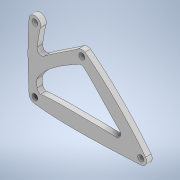
# Autodesk Inventor part: Bracket Concept MK2
Saved by Autodesk Inventor 2021 (Build 250183000, 183)
## iProperties
Created: 2021-05-11
Part Number: Bracket Concept MK2
Material: Generic
Document SubType Name: Modeling
Designer: Jawal
Density: 1 g/cm^3
Appearance: Default
Author: Jawal
Autodesk Inventor part; units mm, degrees
ref_plane "YZ Plane" through (0, 0, 0) normal (1, 0, 0) x (0, 1, 0)
ref_plane "XZ Plane" through (0, 0, 0) normal (0, 1, 0) x (-1, 0, 0)
ref_plane "XY Plane" through (0, 0, 0) normal (0, 0, 1) x (1, 0, 0)
sketch "Sketch1" plane through (0, 0, 0) normal (0, 0, 1) x (1, 0, 0)
  line L0 (-110, 70) -> (110, 70) construction
  line L1 (110, 70) -> (110, -70) construction
  line L2 (110, -70) -> (-110, -70) construction
  line L3 (-110, -70) -> (-110, 70) construction
  circle A0 centre (-90, 55) radius 5
  circle A1 centre (-90, -55) radius 5
  circle A2 centre (90, -55) radius 5
  circle A3 centre (-10, 45) radius 5
  line L4 (-67, 0) -> (-42, 0) construction
  line L5 (-42, 0) -> (-42, -30) construction
  line L6 (-42, -30) -> (-67, -30) construction
  line L7 (-67, -30) -> (-67, 0) construction
  circle A4 centre (-54.5, -11) radius 10 construction
  circle A5 centre (-63.5044, -24.4163) radius 3 construction
  circle A6 centre (-57.3559, -26.4695) radius 3 construction
  circle A7 centre (-51.263, -24.6531) radius 3 construction
  circle A8 centre (-45.3418, -26.5938) radius 3 construction
  arc A9 (-80.8676, 50.9258) -> (-100, 55) centre (-90, 55) ccw
  arc A10 (-4.8937, 53.598) -> (-15.7422, 53.187) centre (-10, 45) ccw
  arc A11 (90.4874, -64.9881) -> (88.2039, -45.1626) centre (90, -55) ccw
  line L8 (-100, 55) -> (-102.0827, 28.5336) construction
  line L9 (-102.0827, 28.5336) -> (-102.0827, 6.1317) construction
  line L10 (-102.0827, 6.1317) -> (-102.0827, -9.3012) construction
  line L11 (-102.0827, -9.3012) -> (-100, -55) construction
  spline S0 degree 4 poles (-100, 55) (-102.0827, 28.5336) (-102.0827, 6.1317) (-102.0827, -9.3012) (-100, -55) knots 1 1 1 1 1 2 2 2 2 2
  line L12 (-80.5098, 51.8478) -> (-81.3111, 50.3761) construction
  line L13 (-33.5621, 40.6884) -> (-15.7422, 53.187) construction
  spline S1 degree 3 poles (-74.3051, 13.1026) (-63.5044, 21.906) (-33.5621, 40.6884) (-15.7422, 53.187) knots 1.047287 1.047287 1.047287 1.047287 2 2 2 2
  line L14 (-90, -65) -> (-53.427, -70) construction
  line L15 (-53.427, -70) -> (0, -70) construction
  line L16 (0, -70) -> (41.9992, -67.3543) construction
  line L17 (41.9992, -67.3543) -> (90.4874, -64.9881) construction
  spline S2 degree 4 poles (-90, -65) (-53.427, -70) (0, -70) (41.9992, -67.3543) (90.4874, -64.9881) knots 1 1 1 1 1 2 2 2 2 2
  arc A12 (-100, -55) -> (-90, -65) centre (-90, -55) ccw
  spline S3 degree 3 poles (-86.2173, -25.9445) (-74.5546, -4.3329) (-47.6722, 13.3107) (-14.3115, 31.1686) knots 1.116691 1.116691 1.116691 1.116691 1.90623 1.90623 1.90623 1.90623
  line L18 (-86.2173, -25.9445) -> (-74.5546, -4.3329) construction
  spline S4 degree 4 poles (-80.5098, 51.8478) (-81.3111, 50.3761) (-83.3432, 41.5365) (-84.547, 29.8741) (-86.4048, 20.3523) knots 1 1 1 1 1 1.500456 1.500456 1.500456 1.500456 1.500456
  spline S5 degree 4 poles (-86.2173, -25.9445) (-87.4499, -31.1305) (-87.0929, -33.8364) (-86.699, -36.6544) (-86.2648, -39.5964) knots 1.850189 1.850189 1.850189 1.850189 1.850189 1.936877 1.936877 1.936877 1.936877 1.936877
  line L19 (-86.2173, -25.9445) -> (-87.4499, -31.1305) construction
  arc A13 (-86.2648, -39.5964) -> (-80.2389, -45.8706) centre (-78.8452, -38.5013) ccw
  line L20 (-87.4499, -31.1305) -> (-87.0929, -33.8364) construction
  line L21 (-87.0929, -33.8364) -> (-86.699, -36.6544) construction
  line L22 (-86.699, -36.6544) -> (-86.2648, -39.5964) construction
  arc A14 (-86.4048, 20.3523) -> (-74.3051, 13.1026) centre (-79.0436, 18.9161) ccw
  line L23 (-81.3111, 50.3761) -> (-83.3432, 41.5365) construction
  line L24 (-83.3432, 41.5365) -> (-84.547, 29.8741) construction
  line L25 (-84.547, 29.8741) -> (-86.4048, 20.3523) construction
  line L26 (-74.3051, 13.1026) -> (-63.5044, 21.906) construction
  line L27 (-63.5044, 21.906) -> (-33.5621, 40.6884) construction
  spline S6 degree 4 poles (-6.0641, 29.79) (10.6281, 14.0219) (25.4029, -2.497) (40.3618, -18.7245) (53.6143, -31.8741) knots 1.041568 1.041568 1.041568 1.041568 1.041568 1.754128 1.754128 1.754128 1.754128 1.754128
  line L28 (-4.8937, 53.598) -> (11.2306, 41.5365) construction
  line L29 (11.2306, 41.5365) -> (41.9992, 15.4144) construction
  line L30 (41.9992, 15.4144) -> (73.02, -16.6008) construction
  line L31 (73.02, -16.6008) -> (98.2566, -49.3583) construction
  spline S7 degree 4 poles (-4.8937, 53.598) (11.2306, 41.5365) (41.9992, 15.4144) (73.02, -16.6008) (98.2566, -49.3583) knots 1 1 1 1 1 2 2 2 2 2
  line L32 (-80.2389, -45.8706) -> (-53.343, -43.1999) construction
  line L33 (-53.343, -43.1999) -> (-23.1335, -44.327) construction
  spline S8 degree 4 poles (-80.2389, -45.8706) (-53.343, -43.1999) (-23.1335, -44.327) (4.8754, -43.9641) (34.4585, -44.2782) (48.1029, -44.6945) knots 1 1 1 1 1 2 2.688212 2.688212 2.688212 2.688212 2.688212
  arc A15 (48.1029, -44.6945) -> (53.6143, -31.8741) centre (48.3317, -37.198) ccw
  line L34 (40.3618, -18.7245) -> (53.6143, -31.8741) construction
  line L35 (-23.1335, -44.327) -> (4.8754, -43.9641) construction
  line L36 (4.8754, -43.9641) -> (34.4585, -44.2782) construction
  line L37 (34.4585, -44.2782) -> (48.1029, -44.6945) construction
  arc A16 (-6.0641, 29.79) -> (-15.1895, 30.6979) centre (-11.2144, 24.338) ccw
  line L38 (-74.5546, -4.3329) -> (-47.6722, 13.3107) construction
  line L39 (-47.6722, 13.3107) -> (-14.3115, 31.1686) construction
  line L40 (-6.0641, 29.79) -> (10.6281, 14.0219) construction
  line L41 (10.6281, 14.0219) -> (25.4029, -2.497) construction
  line L42 (25.4029, -2.497) -> (40.3618, -18.7245) construction
  point P0 (0, 0)
  dimension "d1" = 70
  dimension "d2" = 70
  dimension "d3" = 110
  dimension "d4" = 110
  dimension "d5" = 10
  dimension "d6" = 10
  dimension "d7" = 10
  dimension "d8" = 10
  dimension "d9" = 55
  dimension "d10" = 55
  dimension "d11" = 55
  dimension "d12" = 180
  dimension "d13" = 90
  dimension "d14" = 90
  dimension "d15" = 10
  dimension "d16" = 45
  dimension "d17" = 42
  dimension "d18" = 30
  dimension "d19" = 0
  dimension "d20" = 25
  dimension "d21" = 20
  dimension "d22" = 6
  dimension "d23" = 6
  dimension "d24" = 6
  dimension "d25" = 11
  dimension "d26" = 12.5
  dimension "d27" = 6
  dimension "d28" = 20
  dimension "d29" = 20
  dimension "d30" = 20
  dimension "d37" = 15
  dimension "d38" = 15
  dimension "d41" = 15
  dimension "d42" = 15
  constraints: 22 point on circle, 17 centre point, 16 end point, 4 coincident, 4 parallel, 3 horizontal, 2 midpoint, 2 perpendicular, 2 tangent, 2 vertical, 38 other
  measures "d1" distance from line of point (0, 0) L2
  measures "d2" distance from line of point (0, 0) L0
  measures "d3" distance from line of L1 point (0, 0)
  measures "d4" distance from line of point (0, 0) L3
  measures "d5" diameter of A0
  measures "d6" diameter of A1
  measures "d7" diameter of A2
  measures "d8" diameter of A3
  measures "d9" vertical distance of point (0, 0) A0.centre
  measures "d10" vertical distance of point (0, 0) A1.centre
  measures "d11" vertical distance of A2.centre point (0, 0)
  measures "d12" distance of A2.centre A1.centre
  measures "d13" horizontal distance of point (0, 0) A0.centre
  measures "d14" horizontal distance of point (0, 0) A1.centre
  measures "d15" horizontal distance of point (0, 0) A3.centre
  measures "d16" vertical distance of point (0, 0) A3.centre
  measures "d17" distance from line of point (0, 0) L5
  measures "d18" distance of L4.end L5.end
  measures "d19" distance from line of L4 point (0, 0)
  measures "d20" distance of L5.end L6.end
  measures "d21" diameter of A4
  measures "d22" diameter of A5
  measures "d23" diameter of A6
  measures "d24" diameter of A7
  measures "d25" distance from line of L4 A4.centre
  measures "d26" distance from line of L7 A4.centre
  measures "d27" diameter of A8
  measures "d28" diameter of A9
  measures "d29" diameter of A10
  measures "d30" diameter of A11
  measures "d37" diameter of A13
  measures "d38" diameter of A14
  measures "d41" diameter of A15
  measures "d42" diameter of A16
extrude "Extrusion3" add sketch "Sketch1" along normal blind 9.4 contours S4 A14 S1 A10 S7 A11 S2 A12 S0 A9
equation "\"d1\" = d2"
equation "\"d4\" = d3"
equation "\"d10\" = d9"
equation "\"d11\" = d9"
equation "\"d14\" = d13"
equation "\"d26\" = 0.5 * d20"
body "Solid3"
